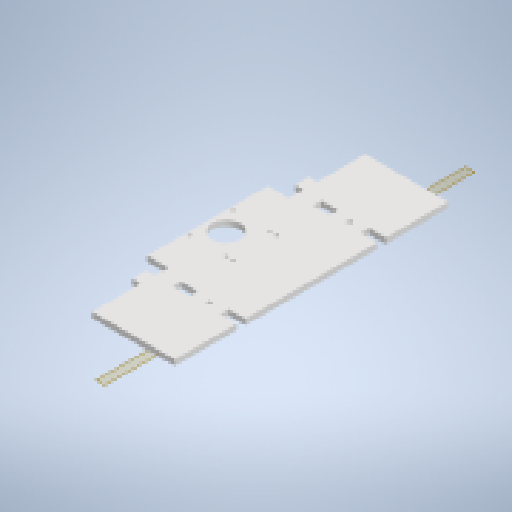
# Autodesk Inventor part: крепление Y
Saved by Autodesk Inventor 2024.2 (Build 282272000, 272)
## iProperties
Created: 2026-02-01
Part Number: крепление Y
Material: Типовые
Document SubType Name: Modeling
Designer: katya_notebook
Density: 1 g/cm^3
Appearance: По умолчанию
Author: katya_notebook
Autodesk Inventor part; units mm, degrees
ref_plane "YZ Plane" through (0, 0, 0) normal (1, 0, 0) x (0, 1, 0)
ref_plane "XZ Plane" through (0, 0, 0) normal (0, 1, 0) x (-1, 0, 0)
ref_plane "РабПлоскость1" through (-53.4845, 288.2505, 354.5129) normal (0, 1, 0) x (-1, 0, 0)
sketch "Эскиз1" plane through (-53.4845, 288.2505, 354.5129) normal (0, 1, 0) x (-1, 0, 0)
  line L0 (45.7889, -56.5016) -> (45.7889, -62.7516) projected
  line L1 (-13.3, 2.5) -> (-13.3, -247.5) projected
  line L2 (-13.3, -220) -> (32.7, -220)
  line L3 (32.7, -220) -> (32.7, -25)
  line L4 (32.7, -25) -> (-13.3, -25)
  line L5 (-13.3, -25) -> (-13.3, -220)
  line L6 (-5.3, -220) -> (142.8907, -220) projected
  line L7 (201.7, -25) -> (166.8907, -25) projected
  point P0 (-53.4845, -354.5129)
  point P1 (-13.3, -25)
  point P2 (-13.3, -220)
  point P3 (32.7, -62.75)
  point P4 (32.7, -56.5)
  constraints: 8 end point, 2 parallel, 2 point on line, 1 horizontal, 1 perpendicular
extrude "Выдавливание1" add sketch "Эскиз1" along normal blind 4
sketch "Эскиз6" plane through (-53.4845, 288.2505, 354.5129) normal (0, -1, 0) x (1, 0, 0)
  line L0 (-32.7, -169.6539) -> (-20.7, -169.6539) projected
  line L1 (-32.7, -175.6539) -> (-32.7, -169.6539) projected
  line L2 (-20.7, -175.6539) -> (-32.7, -175.6539) projected
  line L3 (-20.7, -175.6539) -> (-20.7, -169.6539) projected
  line L4 (-32.7, -69.3164) -> (-20.7, -69.3164) projected
  line L5 (-32.7, -75.3164) -> (-32.7, -69.3164) projected
  line L6 (-20.7, -75.3164) -> (-32.7, -75.3164) projected
  line L7 (-20.7, -75.3164) -> (-20.7, -69.3164) projected
  line L8 (13.3, -220) -> (-32.7, -220) projected
  line L9 (-9.7, -220) -> (-9.7, 17.4543)
  line L10 (13.3, -169.6539) -> (1.3, -169.6539)
  line L11 (13.3, -175.6539) -> (13.3, -169.6539)
  line L12 (1.3, -175.6539) -> (13.3, -175.6539)
  line L13 (1.3, -175.6539) -> (1.3, -169.6539)
  line L14 (13.3, -69.3164) -> (1.3, -69.3164)
  line L15 (13.3, -75.3164) -> (13.3, -69.3164)
  line L16 (1.3, -75.3164) -> (13.3, -75.3164)
  line L17 (1.3, -75.3164) -> (1.3, -69.3164)
  point P0 (53.4845, -354.5129)
  constraints: 18 end point, 8 symmetric about line, 1 midpoint, 1 vertical
extrude "Выдавливание3" cut sketch "Эскиз6" against normal blind 8
sketch "Эскиз7" plane through (-53.4845, 288.2505, 354.5129) normal (0, -1, 0) x (1, 0, 0)
  line L0 (-12.95, -175.6539) -> (-12.95, -169.6539) projected
  line L1 (-7.95, -169.6539) -> (-7.95, -175.6539) projected
  line L2 (-6.45, -175.6539) -> (-6.45, -169.6539) projected
  line L3 (-11.45, -175.6539) -> (-11.45, -169.6539) projected
  line L4 (-12.95, -175.6539) -> (-12.95, -169.6539) projected
  line L5 (-11.45, -175.6539) -> (-7.95, -175.6539)
  line L6 (-7.95, -175.6539) -> (-7.95, -169.6539)
  line L7 (-7.95, -169.6539) -> (-11.45, -169.6539)
  line L8 (-11.45, -169.6539) -> (-11.45, -175.6539)
  circle A0 centre (-9.7, -172.6539) radius 1.75
  line L9 (-32.7, -122.4852) -> (36.9657, -122.4852)
  line L10 (-12.95, -69.3164) -> (-12.95, -75.3164)
  line L11 (-7.95, -75.3164) -> (-7.95, -69.3164)
  line L12 (-6.45, -69.3164) -> (-6.45, -75.3164)
  line L13 (-11.45, -69.3164) -> (-11.45, -75.3164)
  line L14 (-12.95, -69.3164) -> (-12.95, -75.3164)
  line L15 (-11.45, -69.3164) -> (-7.95, -69.3164)
  line L16 (-7.95, -69.3164) -> (-7.95, -75.3164)
  line L17 (-7.95, -75.3164) -> (-11.45, -75.3164)
  line L18 (-11.45, -75.3164) -> (-11.45, -69.3164)
  circle A1 centre (-9.7, -72.3164) radius 1.75
  point P0 (53.4845, -354.5129)
  constraints: 28 end point, 11 symmetric about line, 2 centre point, 2 horizontal, 2 parallel, 2 vertical, 1 perpendicular, 1 tangent, 1 other
extrude "Выдавливание4" cut sketch "Эскиз7" against normal blind 8 contours A0 | A1
sketch "Эскиз8" plane through (-53.4845, 288.2505, 354.5129) normal (0, -1, 0) x (1, 0, 0)
  line L0 (-45.7889, -165.5) -> (-60.7889, -165.5)
  line L1 (-60.7889, -165.5) -> (-60.7889, -79.5)
  line L2 (-60.7889, -79.5) -> (-45.7889, -79.5)
  line L3 (-45.7889, -79.5) -> (-45.7889, -165.5)
  point P0 (53.4845, -354.5129)
  point P1 (-51.7889, -79.5)
  dimension "d15" = 15
  constraints: 8 end point, 2 parallel, 1 horizontal, 1 perpendicular, 1 point on line
  measures "d15" distance of L0.start L0.end
extrude "Выдавливание5" add sketch "Эскиз8" against normal blind 4
sketch "Эскиз9" plane through (-53.4845, 288.2505, 354.5129) normal (0, -1, 0) x (1, 0, 0)
  circle A0 centre (-58.2, -138) radius 1.2645 projected
  circle A1 centre (-58.2, -107) radius 1.2645 projected
  circle A2 centre (-27.2, -107) radius 1.2645 projected
  circle A3 centre (-27.2, -138) radius 1.2645 projected
  point P0 (53.4845, -354.5129)
extrude "Выдавливание6" cut sketch "Эскиз9" against normal blind 4
sketch "Эскиз11" plane through (-86.1845, 288.2505, 329.5129) normal (-1, 0, 0) x (0, 0, 1)
  line L0 (-160.6539, 0) -> (-150.6539, 0)
  line L1 (-150.6539, 0) -> (-150.6539, 4)
  line L2 (-150.6539, 4) -> (-160.6539, 4)
  line L3 (-160.6539, 4) -> (-160.6539, 0)
  line L4 (-44.6539, 4) -> (-34.6539, 4)
  line L5 (-34.6539, 4) -> (-34.6539, 0)
  line L6 (-34.6539, 0) -> (-44.6539, 0)
  line L7 (-44.6539, 0) -> (-44.6539, 4)
  point P0 (-329.5129, -288.2505)
  constraints: 16 end point, 4 parallel, 2 horizontal, 2 perpendicular
ref_plane "РабПлоскость2" through (-105.2734, 252.5455, 159.0129) normal (-1, 0, 0) x (0, 0, 1)
extrude "Выдавливание8" add sketch "Эскиз11" along normal up to surface (19.0889 mm away)
sketch "Эскиз12" plane through (-53.4845, 288.2505, 354.5129) normal (0, -1, 0) x (1, 0, 0)
  line L0 (-60.7889, -79.5) -> (-60.7889, -165.5) projected
  line L1 (-32.7, -220) -> (-32.7, -25) projected
  line L2 (-60.7889, -79.5) -> (-32.7, -79.5)
  line L3 (-32.7, -79.5) -> (-32.7, -165.5)
  line L4 (-32.7, -165.5) -> (-60.7889, -165.5)
  line L5 (-60.7889, -165.5) -> (-60.7889, -79.5)
  point P0 (53.4845, -354.5129)
  point P1 (-32.7, -169.6539)
  point P2 (-32.7, -75.3164)
  point P3 (-32.7, -185.6539)
  dimension "d24" = 86
  constraints: 8 end point, 2 parallel, 1 horizontal, 1 perpendicular, 1 point on line
  measures "d24" distance of L2.end L3.end
extrude "Выдавливание9" add sketch "Эскиз12" against normal blind 4
sketch "Эскиз13" plane through (-53.4845, 288.2505, 354.5129) normal (0, -1, 0) x (1, 0, 0)
  circle A0 centre (-58.2, -107) radius 1.2645 projected
  circle A1 centre (-58.2, -138) radius 1.2645 projected
  circle A2 centre (-42.7, -122.5) radius 3.3 projected
  point P0 (53.4845, -354.5129)
extrude "Выдавливание10" cut sketch "Эскиз13" against normal blind 8
sketch "Эскиз14" plane through (-53.4845, 288.2505, 354.5129) normal (0, -1, 0) x (1, 0, 0)
  line L0 (-45.7603, -165.5) -> (-45.7603, -175.6539)
  line L1 (-45.7603, -175.6539) -> (-32.7, -175.6539)
  line L2 (-45.7603, -185.6539) -> (-32.7, -185.6539)
  line L3 (-32.7, -185.6539) -> (-32.7, -220)
  line L4 (-32.7, -220) -> (-45.7603, -220)
  line L5 (-45.7603, -220) -> (-45.7603, -185.6539)
  line L6 (-45.7603, -79.5) -> (-45.7603, -69.6539)
  line L7 (-45.7603, -59.6539) -> (-45.7603, -25)
  line L8 (-45.7603, -25) -> (-32.7, -25)
  line L9 (-32.7, -79.5) -> (-45.7603, -79.5)
  line L10 (-45.7603, -79.5) -> (-45.7603, -69.6539)
  line L11 (-45.7603, -25) -> (-32.7, -25)
  line L12 (-32.7, -25) -> (-32.7, -59.6539)
  line L13 (-32.7, -59.6539) -> (-45.7603, -59.6539)
  line L14 (-45.7603, -59.6539) -> (-45.7603, -25)
  line L15 (-45.7603, -79.5) -> (-32.7, -79.5)
  line L16 (-32.7, -79.5) -> (-32.7, -69.6539)
  line L17 (-32.7, -69.6539) -> (-45.7603, -69.6539)
  line L18 (-45.7603, -69.6539) -> (-45.7603, -79.5)
  line L19 (-45.7603, -175.6539) -> (-32.7, -175.6539)
  line L20 (-32.7, -175.6539) -> (-32.7, -165.5)
  line L21 (-32.7, -165.5) -> (-45.7603, -165.5)
  line L22 (-45.7603, -165.5) -> (-45.7603, -175.6539)
  point P0 (53.4845, -354.5129)
  point P1 (13.3, -220)
  point P2 (-32.7, -25)
  point P3 (-45.7603, -69.6539)
  point P4 (-45.7603, -165.5)
  constraints: 46 end point, 8 parallel, 4 horizontal, 4 perpendicular, 3 point on line
extrude "Выдавливание11" add sketch "Эскиз14" against normal blind 4
sketch "Эскиз16" plane through (-53.4845, 288.2505, 354.5129) normal (0, -1, 0) x (1, 0, 0)
  circle A0 centre (-42.7, -122.5) radius 4.1 projected
  circle A1 centre (-47.7, -122.5) radius 10
  circle A2 centre (-58.2, -107) radius 1.2645 projected
  circle A3 centre (-27.2, -107) radius 1.2645 projected
  circle A4 centre (-27.2, -138) radius 1.2645 projected
  circle A5 centre (-58.2, -138) radius 1.2645 projected
  circle A6 centre (-63.2, -107) radius 1.2645
  circle A7 centre (-32.2, -107) radius 1.2645
  circle A8 centre (-63.2, -138) radius 1.2645
  circle A9 centre (-32.2, -138) radius 1.2645
  point P0 (53.4845, -354.5129)
  dimension "d35" = 5
  dimension "d36" = 0
  dimension "d37" = 20
  dimension "d38" = 5
  dimension "d39" = 5
  dimension "d40" = 5
  dimension "d41" = 5
  constraints: 5 centre point, 4 equal radius
  measures "d35" distance of A0.centre A1.centre
  measures "d36" vertical distance of A0.centre A1.centre
  measures "d37" diameter of A1
  measures "d38" distance of A2.centre A6.centre
  measures "d39" distance of A5.centre A8.centre
  measures "d40" distance of A4.centre A9.centre
  measures "d41" distance of A3.centre A7.centre
extrude "Выдавливание13" cut sketch "Эскиз16" against normal blind 10 contours A0 | A1 | A6 | A7 | A8 | A9
